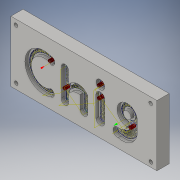
# Autodesk Inventor part: NewNameChirag
Saved by Autodesk Inventor 2016 (Build 200138000, 138)
## iProperties
Created: 2016-09-23
Part Number: NewNameChirag
Material: Generic
Document SubType Name: Modeling
Designer: Shaan Sharma
Density: 1 g/cm^3
Appearance: Default
Author: Shaan Sharma
Autodesk Inventor part; units mm, degrees
ref_plane "YZ Plane" through (0, 0, 0) normal (1, 0, 0) x (0, 1, 0)
ref_plane "XZ Plane" through (0, 0, 0) normal (0, 1, 0) x (-1, 0, 0)
ref_plane "XY Plane" through (0, 0, 0) normal (0, 0, 1) x (1, 0, 0)
sketch "Sketch1" plane through (0, 0, 0) normal (0, 0, 1) x (1, 0, 0)
  line L0 (-174.625, 111.125) -> (130.175, 111.125)
  line L1 (130.175, 111.125) -> (130.175, -15.875)
  line L2 (130.175, -15.875) -> (-174.625, -15.875)
  line L3 (-174.625, -15.875) -> (-174.625, 111.125)
  point P0 (0, 0)
  dimension "d0" = 127
  dimension "d1" = 304.8
  constraints: 8 end point, 2 parallel, 1 horizontal, 1 perpendicular
  measures "d0" distance of L2.end L0.start
  measures "d1" distance of L1.end L2.end
extrude "Extrusion1" add sketch "Sketch1" along normal blind 25.4
sketch "Sketch2" plane through (0, 0, 25.4) normal (0, 0, 1) x (1, 0, 0)
  arc A0 (-89.9147, 65.1281) -> (-91.28, 21.8576) centre (-105.641, 43.9675) ccw
  arc A1 (-91.3052, 80.8519) -> (-91.28, 7.0928) centre (-105.641, 43.9675) ccw
  arc A2 (-91.28, 7.0928) -> (-91.28, 21.8576) centre (-91.28, 14.4752) ccw
  arc A3 (-89.9147, 65.1281) -> (-91.3052, 80.8519) centre (-90.6099, 72.99) ccw
  line L0 (-69.1328, 16.3208) -> (-69.1328, 73.5344)
  line L1 (-54.368, 16.3208) -> (-54.368, 73.5344)
  arc A4 (-69.1328, 16.3208) -> (-54.368, 16.3208) centre (-61.7504, 14.4752) ccw
  arc A5 (-54.368, 73.5344) -> (-69.1328, 73.5344) centre (-61.7504, 73.5344) ccw
  arc A6 (-14.0573, 29.8688) -> (-54.368, 30.9892) centre (-34.5504, 18.2752) ccw
  arc A7 (-13.7648, 47.696) -> (-54.368, 47.696) centre (-34.0664, 34.6261) ccw
  line L2 (-14.0573, 29.8688) -> (-14.0573, 14.2776)
  line L3 (-14.0573, 48.1396) -> (-14.0573, 29.8688)
  line L4 (-30.3752, 14.2776) -> (-30.3752, 58.4872)
  arc A8 (-30.3752, 14.2776) -> (-14.0573, 14.2776) centre (-22.2162, 15.2758) ccw
  line L5 (2.8456, 15.2758) -> (2.8456, 58.4872)
  line L6 (21.3017, 15.2758) -> (21.3017, 58.4872)
  arc A9 (2.8456, 15.2758) -> (21.3017, 15.2758) centre (12.0736, 16.3458) ccw
  arc A10 (21.3017, 58.4872) -> (2.8456, 58.4872) centre (12.0736, 58.4872) ccw
  circle A11 centre (12.0736, 80.9168) radius 9.228
  circle A12 centre (68.1313, 53.8586) radius 21.2102
  circle A13 centre (68.1313, 53.8586) radius 8.0022
  arc A14 (49.3965, 3.6206) -> (89.1971, 33.323) centre (58.2137, 33.323) ccw
  line L7 (89.1971, 33.323) -> (89.1971, 51.3872)
  arc A15 (49.9069, 21.9732) -> (67.3833, 32.6616) centre (53.1362, 36.3249) ccw
  arc A16 (49.9069, 21.9732) -> (49.3965, 3.6206) centre (47.8533, 12.8469) ccw
  point P0 (0, 0)
  dimension "d42" = 13.208
  dimension "d43" = 13.208
  constraints: 32 point on circle, 17 centre point, 16 end point, 8 vertical, 5 tangent, 2 point on line, 1 coincident, 1 concentric
  measures "d42" radial gap between concentric circles of A1 A0
  measures "d43" radial gap between concentric circles of A12 A13
emboss "Emboss1" sketch "Sketch2" operation cut depth 6.35 direction (0, 0, -1)
hole "Hole1" at (-163.3305, -4.0099, 25.4) direction (0, 0, -1) diameter 7.62 end through all
hole "Hole2" at (-163.7335, 100.3697, 25.4) direction (0, 0, -1) diameter 7.62 end through all
hole "Hole3" at (117.1647, 99.5637, 25.4) direction (0, 0, -1) diameter 7.62 end through all
hole "Hole4" at (117.5677, -6.025, 25.4) direction (0, 0, -1) diameter 7.62 end through all
body "Solid1"
